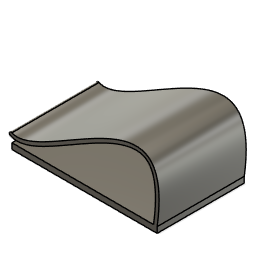
Clipsi v1 (Autodesk Fusion 360 design; units mm, degrees)
Autodesk Fusion 360 part; units mm, degrees
sketch "Sketch1" plane through (0, 0, 0) normal (0, 0, 1) x (1, 0, 0)
  line L0 (0, 0) -> (-50, 0)
  line L1 (0, 0) -> (0, 2)
  line L2 (-1.3, 2) -> (-50, 2)
  line L3 (-50, 2) -> (-50, 0)
  spline S0 degree 5 poles (0, 2) (0.2307, 3.6309) (0.5907, 6.7318) (0.8261, 10.9001) (0.5267, 15.4851) (-0.8852, 19.5674) (-3.3339, 21.9932) (-6.7796, 22.8075) (-11.116, 22.1482) (-16.1407, 20.2893) (-21.5902, 17.5915) (-27.1703, 14.4591) (-32.5849, 11.2992) (-37.566, 8.4811) (-41.901, 6.3001) (-45.4722, 4.9237) (-47.6857, 4.5168) (-48.9829, 4.6062) (-49.6876, 4.8397) (-50, 5) knots 0 0 0 0 0 0 0.066667 0.133333 0.2 0.266667 0.333333 0.4 0.466667 0.533333 0.6 0.666667 0.733333 0.8 0.866667 0.933333 1 1 1 1 1 1
  spline S1 degree 3 poles (-1.2131, 2.1716) (-0.4467, 7.589) (-0.3795, 11.8865) (-0.956, 14.9516) (-1.3978, 17.3005) (-2.2014, 18.8822) (-3.2428, 19.8441) (-4.1747, 20.7048) (-5.3307, 21.147) (-6.8853, 21.2107) (-8.9772, 21.2965) (-11.755, 20.5984) (-14.8645, 19.3312) (-19.5062, 17.4395) (-24.856, 14.3533) (-29.7999, 11.5084) (-33.6405, 9.2984) (-37.2256, 7.255) (-40.2595, 5.8203) (-43.0437, 4.5037) (-45.3612, 3.6749) (-47.2994, 3.4598) (-48.5149, 3.325) (-49.6177, 3.4268) (-50.5593, 3.91) knots 0 0 0 0 0.134766 0.134766 0.134766 0.238042 0.238042 0.238042 0.330458 0.330458 0.330458 0.454818 0.454818 0.454818 0.640456 0.640456 0.640456 0.784666 0.784666 0.784666 0.917008 0.917008 0.917008 1 1 1 1
  arc A0 (-50, 5) -> (-50.5593, 3.91) centre (-50.2797, 4.455) ccw
  line L4 (-1.2131, 2.1716) -> (-1.3, 2)
  point P0 (-6.9382, 22.4385)
  point P1 (-38.6769, 7.9716)
  dimension "d1" = 50
  dimension "d2" = 2
  dimension "d3" = -1.2252
  constraint coincident L0.start L1.start
  constraint horizontal L0
  constraint perpendicular L0 L1
  constraint perpendicular L1 L2
  constraint perpendicular L0 L3
  measures "d1" distance of L0.start L0.end
  measures "d2" distance of L0.start L1.end
extrude "Extrude1" add sketch "Sketch1" along normal blind 30
